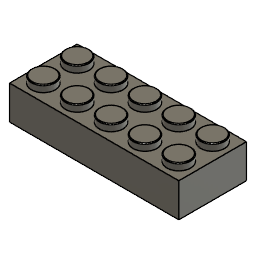
lego_brick (Autodesk Fusion 360 design; units mm, degrees)
part number: 2026-05-19-17-16-54-995
Autodesk Fusion 360 part; units mm, degrees
sketch "Boceto1" plane through (0, 0, 0) normal (0, 1, 0) x (1, 0, 0)
  line L0 (25, 10) -> (0, 10)
  line L1 (0, 10) -> (0, 0)
  line L2 (0, 0) -> (25, 0)
  line L3 (25, 0) -> (25, 10)
  dimension "d10" = 25
  dimension "d11" = 10
  constraint horizontal L0
  constraint vertical L1
  constraint horizontal L2
  constraint vertical L3
  constraint coincident L1.end L2.start
  measures "d10" distance of L0.start L0.end
  measures "d11" distance of L0.start L2.end
extrude "Extruir1" add sketch "Boceto1" along normal blind 5
shell "Vaciado1" thickness 0.3 removed faces 1 at (8.3333, 0, -6.6667)
sketch "Boceto2" plane through (0, 5, 0) normal (0, 1, 0) x (-1, 0, 0)
  line L0 (-25, 0) -> (-25, -10)
  line L1 (-25, -10) -> (0, -10)
  line L2 (0, -10) -> (0, 0)
  line L3 (0, 0) -> (-25, 0)
  circle A0 centre (-2.5, -2.5) radius 1.75
  dimension "d15" = 3.5
  dimension "d16" = 2.5
  dimension "d17" = 2.5
  measures "d15" diameter of A0
  measures "d16" vertical distance of L2.end A0.centre
  measures "d17" horizontal distance of L2.end A0.centre
extrude "Extruir2" add sketch "Boceto2" along normal blind 1 contours A0
fillet "Empalme1" radius 0.1 1 edges at (4.1316, 6, -3.1328)
pattern_linear "Patrón R1" count 5 spacing 5 along (1, 0, 0) count 2 spacing 5 along (0, 0, -1) of "Extruir2", "Empalme1"
equation "height = 5 mm"
equation "width = 5 mm"
equation "length = 5 mm"
equation "horizontal_studs = 2"
equation "vertical_studs = 5"
equation "stud_height = 1 mm"
equation "stud_diameter = 3.5 mm"
equation "stud_fillet = 0.1 mm"
equation "shell = 0.3 mm"
equation "d10 = length * vertical_studs"
equation "d11 = width * horizontal_studs"
equation "d12 = height"
equation "d14 = shell"
equation "d15 = stud_diameter"
equation "d16 = length / 2"
equation "d17 = width / 2"
equation "d18 = stud_height"
equation "d21 = stud_fillet"
equation "d22 = vertical_studs"
equation "d23 = horizontal_studs"
equation "d24 = width"
equation "d25 = length * -1"
